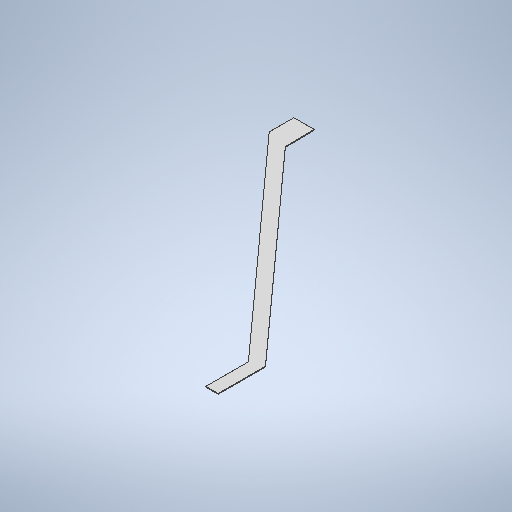
# Autodesk Inventor part: BSH 025 rib board cone
Saved by Autodesk Inventor 2025 (Build 290162010, 162A)
## iProperties
Created: 2024-07-23
Part Number: BSH 025 rib board cone
Material: 09g2s
Document SubType Name: Sheet Metal
Designer: pokla
Stock Number: БШК 022 шпангоут борт
Mass: 4739.97 g
Surface Area: 4201.54 cm^2
Volume: 603.817 cm^3
Density: 7.85 g/cm^3
Sheet Metal Rule: AISI304 3mm Die 32
Sheet Metal Width: 0,000 mm
Sheet Metal Length: 0,000 mm
Sheet Metal Area: 0,000 mm^2
Appearance: Default
Author: admin
Autodesk Inventor part; units mm, degrees
ref_plane "YZ Plane" through (0, 0, 0) normal (1, 0, 0) x (0, 1, 0)
ref_plane "XZ Plane" through (0, 0, 0) normal (0, 1, 0) x (-1, 0, 0)
ref_plane "XY Plane" through (0, 0, 0) normal (0, 0, 1) x (1, 0, 0)
sketch "Sketch1" plane through (0, 0, 0) normal (0, 0, 1) x (1, 0, 0)
  line L0 (1200, 2950) -> (-1200, 2950)
  line L1 (-1200, 2950) -> (-1200, 0)
  line L2 (-1200, 0) -> (1200, 0)
  line L3 (1200, 0) -> (1200, 2950)
  line L4 (1150, 2950) -> (1150, 0)
  line L5 (-1150, 0) -> (-1150, 2950) construction
  line L6 (0, 2950) -> (0, 50) construction
  line L7 (-1100, 200) -> (-950, 50)
  line L8 (-1200, 100) -> (-1100, 100)
  line L9 (-1100, 100) -> (-1100, 0)
  line L10 (-1100, 200) -> (-1150, 2950)
  arc A0 (-1100.4545, 224.9959) -> (-1082.3223, 182.3223) centre (-1100, 200) ccw
  arc A1 (-1082.3223, 182.3223) -> (-1100.4545, 224.9959) centre (-1100, 200) ccw construction
  line L11 (-1200, 255) -> (-1101, 255) construction
  line L12 (0, 50) -> (-950, 50)
  line L13 (0, 50) -> (0, 0)
  line L14 (1505.3449, -225.894) -> (355.3449, -225.894)
  line L15 (-1200, 245) -> (-1100.8182, 245)
  line L16 (-1200, 2900) -> (-1149.0909, 2900)
  line L17 (-1115.5511, 1055.3131) -> (-385.5, 244.8343)
  line L18 (-1200, 1174.3582) -> (-1117.7156, 1174.3582)
  line L19 (-385.5, 0) -> (-385.5, 244.8343)
  line L20 (-435.5, 0) -> (-435.5, 300.3427)
  line L21 (-1200, 1074.3582) -> (-385.5, 170.1271)
  line L22 (-435.5, 53) -> (-385.5, 53)
  line L23 (-1200, 245) -> (-101.8902, 245)
  point P0 (-435.5, 225.6354)
  point P1 (-435.5, 50)
  point P2 (-385.5, 50)
  dimension "d3" = 2400
  dimension "d4" = 2950
  dimension "d5" = 50
  dimension "d6" = 100
  dimension "d7" = 50
  dimension "d9" = 135
  dimension "d10" = 950
  dimension "d11" = 1150
  dimension "d12" = 136.042
  dimension "d13" = 50
  dimension "d14" = 100
  dimension "d15" = 212.132
  dimension "d17" = 55
  dimension "d20" = 200
  dimension "d50" = 2705
  dimension "d53" = 50
  dimension "d55" = 1895
  dimension "d57" = 100
  dimension "d59" = 385.5
  dimension "d60" = 50
  dimension "d62" = 50
  dimension "d63" = 3
  dimension "d64" = 244.8343
  measures "d3" distance of L3.start L1.end
  measures "d4" distance of L1.end L1.start
  measures "d5" diameter of A0
  measures "d6" distance of L8.start L8.end
  measures "d7" distance between parallel lines of L1 L5
  measures "d9" angle of L12 L7
  measures "d10" distance of L6.end L7.end
  measures "d11" distance of L14.start L14.end
  measures "d12" angle of L7 L10
  measures "d13" distance between parallel lines of L2 L12
  measures "d14" distance from line of L1 L10.start
  measures "d15" distance of L10.start L7.end
  measures "d17" vertical distance of L10.start L11.end
  measures "d20" distance from line of L2 A1.centre
  measures "d50" distance of L1.start L15.start
  measures "d53" distance of L16.start L1.start
  measures "d55" distance of L10.end L17.start
  measures "d57" distance of L21.start L18.start
  measures "d59" distance of L19.start point (0, 0)
  measures "d60" distance between parallel lines of L20 L19
  measures "d62" distance between parallel lines of L21 L17
  measures "d63" distance between parallel lines of L12 L22
  measures "d64" distance of L19.start L17.end
extrude "Plate1" add sketch "Sketch1" along normal blind 3 contours L10 L21 L1 L18 | L17 L20 L23 L21 L10 | L17 L23 L20 | L22 L20 L21 L19 | L23 L20 L21 | L17 L19 L21 L20 L23
equation "\"d11\" = d10 + d18"
equation "\"d14\" = d6"
equation "\"d2\" = Thickness"
equation "\"BendReliefWidth\" = Thickness"
equation "\"BendReliefDepth\" = 0.5 * Thickness"
equation "\"CornerReliefSize\" = 4 * Thickness"
equation "\"MinimumRemnant\" = 2 * Thickness"
equation "\"TransitionRadius\" = BendRadius"
equation "\"JacobiRadiusSize\" = BendRadius"
equation "\"GapSize\" = Thickness"
equation "\"d18\" = d19"
equation "\"Thickness\" = 3"
equation "\"BendRadius\" = 5"
equation "\"d19\" = 200"
body "Solid1"
